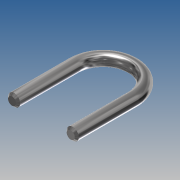
# Autodesk Inventor part: DD_KVD_002_14
Saved by Autodesk Inventor 2017.3 (Build 213256000, 256)
## iProperties
Created: 2023-12-14
Part Number: DD_KVD_002_14
Material: Nerezová ocel
Document SubType Name: Modeling
Designer: Darena
Manufacturer: Standard
Standards Organization: Custom
Density: 8 g/cm^3
Appearance: Pololeštěná
Author: Darena
Autodesk Inventor part; units mm, degrees
ref_plane "YZ Plane" through (0, 0, 0) normal (1, 0, 0) x (0, 1, 0)
ref_plane "XZ Plane" through (0, 0, 0) normal (0, 1, 0) x (-1, 0, 0)
ref_plane "XY Plane" through (0, 0, 0) normal (0, 0, 1) x (1, 0, 0)
sketch "Náčrt5" plane through (0, 0, 0) normal (1, 0, 0) x (0, 1, 0)
  circle A0 centre (0, 0) radius 3
  dimension "d23" = 6
  constraints: 1 centre point, 1 coincident
  measures "d23" diameter of A0
sketch "Náčrt6" plane through (0, 0, 0) normal (0, 0, 1) x (1, 0, 0)
  line L0 (-14.5, -45) -> (-14.5, -14.5)
  line L1 (0, 0) -> (0, 0)
  line L2 (14.5, -14.5) -> (14.5, -45)
  line L3 (-14.5, -45) -> (14.5, -45) construction
  arc A0 (0, 0) -> (-14.5, -14.5) centre (0, -14.5) ccw
  arc A1 (14.5, -14.5) -> (0, 0) centre (0, -14.5) ccw
  point P0 (0, 0)
  point P1 (14.5, 0)
  point P2 (0, 0)
  dimension "d46" = 29
  dimension "d47" = 45
  dimension "d48" = 14.5
  constraints: 8 end point, 4 point on circle, 4 tangent, 2 centre point, 2 perpendicular, 2 point on line, 1 coincident, 1 concentric, 1 midpoint, 1 parallel, 1 vertical
  measures "d46" distance between parallel lines of L2 L0
  measures "d47" distance of point (14.5, 0) L2.end
  measures "d48" radius of A0
sweep "Tažení4" add profiles "Náčrt5" path "Náčrt6"
chamfer "Zkosení4" distance 1 angle 45 5 edges at (-11.5, -45, 0) (-11.5, -14.5, 0) (0, -3, 0) (11.5, -14.5, 0) (11.5, -45, 0)
equation "\"d48\" = 0.5 * d46"
